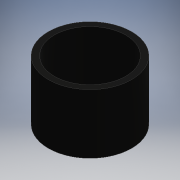
# Autodesk Inventor part: オイレス　12-14 8
Saved by Autodesk Inventor 2016 (Build 200138000, 138)
## iProperties
Created: 2019-03-07
Part Number: オイレス　12-14 8
Material: アセタール樹脂、黒
Document SubType Name: Modeling
Designer: mozar
Density: 1.425 g/cm^3
Appearance: 滑らか - 黒
Mass: 0.58198 g
Surface Area: 8.98495 cm^2
Volume: 0.408407 cm^3
Author: mozar
Autodesk Inventor part; units mm, degrees
ref_plane "YZ Plane" through (0, 0, 0) normal (1, 0, 0) x (0, 1, 0)
ref_plane "XZ Plane" through (0, 0, 0) normal (0, 1, 0) x (-1, 0, 0)
ref_plane "XY Plane" through (0, 0, 0) normal (0, 0, 1) x (1, 0, 0)
sketch "スケッチ1" plane through (0, 0, 0) normal (0, 0, 1) x (1, 0, 0)
  circle A0 centre (0, 0) radius 7
  circle A1 centre (0, 0) radius 6
  dimension "d0" = 14
  dimension "d1" = 12
  constraints: 2 centre point, 2 coincident
  measures "d0" diameter of A0
  measures "d1" diameter of A1
extrude "押し出し1" add sketch "スケッチ1" along normal blind 10
